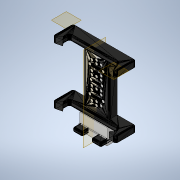
# Autodesk Inventor part: e4-phone_1piece pivot 2019
Saved by Autodesk Inventor 2020 (Build 240168000, 168)
## iProperties
Created: 2019-01-02
Part Number: e4-phone_1piece pivot 2019
Material: Generic
Document SubType Name: Modeling
Designer: ball
Density: 1 g/cm^3
Appearance: Default
Author: ball
Autodesk Inventor part; units mm, degrees
ref_plane "YZ Plane" through (0, 0, 0) normal (1, 0, 0) x (0, 1, 0)
ref_plane "XZ Plane" through (0, 0, 0) normal (0, 1, 0) x (-1, 0, 0)
ref_plane "Work Plane1" through (-89.882, 196577.8405, 29.6599) normal (0, 0, -1) x (-1, 0, 0)
ref_plane "Work Plane4" through (-3, 0, 29.6599) normal (0, 1, 0) x (1, 0, 0)
ref_plane "Work Plane5" through (-102.2297, 0, 0) normal (0, 1, 0) x (1, 0, 0)
sketch "Sketch9" plane through (-27.41, -83, 0) normal (0, 0, -1) x (-1, 0, 0)
  line L0 (-24.41, -8) -> (61.8197, -8) construction
  line L1 (-1.9451, -8) -> (-1.9451, -26) construction
  line L2 (39.3549, -26) -> (39.3549, -8) construction
  line L3 (0.0549, -28) -> (37.3549, -28) construction
  line L4 (-1.9451, -8) -> (39.3549, -8)
  line L5 (39.3549, -8) -> (39.3549, -30)
  line L6 (-1.9451, -30) -> (-1.9451, -8)
  line L7 (-1.9451, -30) -> (39.3549, -30)
  point P0 (-27.41, 83)
  dimension "d50" = 2
  constraints: 8 end point, 2 parallel, 1 horizontal, 1 perpendicular
  measures "d50" distance between parallel lines of L3 L7
extrude "Extrusion5" add sketch "Sketch9" against normal blind 17.12
sketch "Sketch12" plane through (-27.41, -83, 17.12) normal (0, 0, 1) x (1, 0, 0)
  line L0 (1.9451, -8) -> (-39.3549, -8) construction
  line L1 (1.9451, -30) -> (1.9451, -8) construction
  line L2 (1.9451, -21.9992) -> (-39.4839, -21.9992) construction
  line L3 (-39.3549, -8) -> (-39.3549, -30) projected
  line L4 (-39.3549, -8) -> (1.9451, -8)
  line L5 (1.9451, -8) -> (1.9451, -21.9992)
  line L6 (1.9451, -21.9992) -> (-39.3549, -21.9992)
  line L7 (-39.3549, -21.9992) -> (-39.3549, -8)
  point P0 (27.41, 83)
  constraints: 10 end point, 2 parallel, 2 perpendicular, 1 horizontal, 1 point on line
extrude "Extrusion6" cut sketch "Sketch12" against normal blind 1.524
sketch "Sketch13" plane through (-27.41, -83, 0) normal (0, 0, -1) x (-1, 0, 0)
  line L0 (39.3549, -30) -> (-1.9451, -30) projected
  line L1 (39.3549, -8) -> (39.3549, -30) projected
  line L2 (-1.9451, -30) -> (39.3549, -30)
  line L3 (39.3549, -30) -> (39.3549, -22)
  line L4 (39.3549, -22) -> (-1.9451, -22)
  line L5 (-1.9451, -22) -> (-1.9451, -30)
  point P0 (-27.41, 83)
  dimension "d55" = 8
  constraints: 8 end point, 2 parallel, 1 horizontal, 1 perpendicular, 1 point on line
  measures "d55" distance of L3.end L2.end
extrude "Extrusion7" cut sketch "Sketch13" against normal blind 1.524
ref_plane "Work Plane3" through (-46.1149, -8, 26.5711) normal (1, 0, 0) x (0, 0, -1)
sketch "Sketch14" plane through (-35.8127, -28.3817, 11.8) normal (0, 0, 1) x (1, 0, 0)
  circle A0 centre (-10.2977, 6.8817) radius 2.0002 construction
  circle A1 centre (-10.2977, -2.3243) radius 2
  line L0 (-10.2977, -2.3243) -> (-10.2977, -29.2737) construction
  circle A2 centre (-10.2977, -29.2737) radius 2
  point P0 (35.8127, 28.3817)
  dimension "d58" = 4
  dimension "d59" = 26.9494
  dimension "d60" = 4
  constraints: 2 centre point, 2 end point, 1 coincident, 1 vertical
  measures "d58" diameter of A1
  measures "d59" distance of L0.start L0.end
  measures "d60" diameter of A2
sketch "Sketch15" plane through (-35.8127, -28.3817, 11.8) normal (0, 0, 1) x (1, 0, 0)
  line L0 (-25.4123, 17.2723) -> (3.8236, 17.2723)
  line L1 (3.8236, 17.2723) -> (3.8236, -49.3954)
  line L2 (3.8236, -49.3954) -> (-25.4123, -49.3954)
  line L3 (-25.4123, -49.3954) -> (-25.4123, 17.2723)
  point P0 (35.8127, 28.3817)
  constraints: 8 end point, 2 parallel, 1 horizontal, 1 perpendicular
extrude "Extrusion8" add sketch "Sketch15" against normal blind 12
extrude "Extrusion9" cut sketch "Sketch14" against normal blind 30
body "Solid2"
